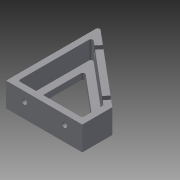
# Autodesk Inventor part: lcd_halterung_162C_links
Saved by Autodesk Inventor 2015 (Build 190159000, 159)
## iProperties
Created: 2014-11-18
Part Number: lcd_halterung_162C_links
Material: Generisch
Document SubType Name: Modeling
Designer: Zephram
Density: 1 g/cm^3
Appearance: Vorgabe
Author: Zephram
Autodesk Inventor part; units mm, degrees
ref_plane "YZ Plane" through (0, 0, 0) normal (1, 0, 0) x (0, 1, 0)
ref_plane "XZ Plane" through (0, 0, 0) normal (0, 1, 0) x (-1, 0, 0)
ref_plane "XY Plane" through (0, 0, 0) normal (0, 0, 1) x (1, 0, 0)
sketch "Skizze1" plane through (0, 0, 0) normal (0, 0, 1) x (1, 0, 0)
  line L0 (0, 0) -> (0, 46.8858)
  line L1 (0, 46.8858) -> (38, 15)
  line L2 (38, 15) -> (38, 0)
  line L3 (38, 0) -> (0, 0)
  line L4 (6.5, 32.9465) -> (6.5, 6.5)
  line L5 (6.5, 6.5) -> (31.5, 6.5)
  line L6 (31.5, 6.5) -> (31.5, 11.969)
  line L7 (31.5, 11.969) -> (6.5, 32.9465)
  dimension "d0" = 130
  dimension "d1" = 15
  dimension "d2" = 38
  dimension "d3" = 6.5
  dimension "d4" = 6.5
  dimension "d5" = 6.5
  dimension "d6" = 6.5
  constraints: 16 end point, 5 parallel, 1 perpendicular, 1 vertical
  measures "d0" angle of L2 L1
  measures "d1" distance of L1.end L2.end
  measures "d2" distance of L2.end L0.start
  measures "d3" distance between parallel lines of L3 L5
  measures "d4" distance between parallel lines of L0 L4
  measures "d5" distance between parallel lines of L1 L7
  measures "d6" distance between parallel lines of L2 L6
extrude "Extrusion1" add sketch "Skizze1" along normal blind 12
sketch "Skizze2" plane through (0, 0, 12) normal (0, 0, 1) x (1, 0, 0)
  line L0 (3, 40.4523) -> (3, 3)
  line L1 (3, 3) -> (35, 3)
  line L2 (35, 3) -> (35, 13.6011)
  line L3 (35, 13.6011) -> (3, 40.4523)
  line L4 (0, 0) -> (38, 0) projected
  line L5 (0, 46.8858) -> (0, 0) projected
  line L6 (38, 15) -> (0, 46.8858) projected
  line L7 (38, 0) -> (38, 15) projected
  dimension "d9" = 3
  dimension "d10" = 3
  dimension "d11" = 3
  dimension "d12" = 3
  constraints: 8 end point, 4 parallel, 1 horizontal, 1 perpendicular
  measures "d9" distance between parallel lines of L6 L3
  measures "d10" distance between parallel lines of L5 L0
  measures "d11" distance between parallel lines of L4 L1
  measures "d12" distance between parallel lines of L7 L2
extrude "Extrusion2" cut sketch "Skizze2" against normal blind 9 contours L3 L2 L1 L0
sketch "Skizze3" plane through (3, 3, 12) normal (0, 1, 0) x (1, 0, 0)
  line L0 (-3, 0) -> (-3, 12) projected
  line L1 (-3, 12) -> (35, 12) projected
  line L2 (35, 12) -> (35, 0) projected
  line L3 (35, 0) -> (32, 0) projected
  line L4 (32, 0) -> (0, 0) projected
  line L5 (0, 0) -> (-3, 0) projected
  line L6 (32, 0) -> (32, 9) projected
  line L7 (32, 9) -> (0, 9) projected
  line L8 (0, 9) -> (0, 0) projected
  line L9 (0, 0) -> (0, 9) projected
  line L10 (32, 0) -> (32, 9) projected
  line L11 (32, 4.5) -> (0, 4.5)
  point P0 (6, 4.5)
  point P1 (26, 4.5)
  dimension "d15" = 6
  dimension "d17" = 6
  constraints: 2 end point, 2 midpoint, 2 point on line
  measures "d15" distance of point (6, 4.5) L11.end
  measures "d17" distance of point (26, 4.5) L11.start
hole "Bohrung1" at (9, 3, 7.5) at (29, 3, 7.5) direction (0, -1, 0) diameter 2.7 depth 8 tip angle 118
fillet "Rundung1" radius 1 9 edges at (35, 13.6011, 7.5) (31.5, 11.969, 1.5) (31.5, 6.5, 1.5) (35, 3, 7.5) (6.5, 6.5, 1.5) (3, 3, 7.5) (6.5, 32.9465, 1.5) (3, 40.4523, 7.5) (0, 46.8858, 6)
sketch "Skizze4" plane through (4.6428, 39.0738, 3) normal (-0.6427876, -0.7660444, 0) x (0.7660444, -0.6427876, 0)
  line L0 (-6.0607, 9) -> (0, 9) projected
  line L1 (0, 9) -> (39.1622, 9) projected
  line L2 (39.1622, 9) -> (43.5447, 9) projected
  line L3 (43.5447, 9) -> (43.5447, -3) projected
  line L4 (43.5447, -3) -> (-6.0607, -3) projected
  line L5 (-6.0607, -3) -> (-6.0607, 9) projected
  line L6 (0, 0) -> (0, 9) projected
  line L7 (0, 0) -> (39.1622, 0) projected
  line L8 (39.1622, 0) -> (39.1622, 9) projected
  point P0 (21.5596, -3)
  point P1 (35.1622, 6.5)
  point P2 (4.1622, 6.5)
  point P3 (35.1622, 6.5)
  dimension "d26" = 2.5
  dimension "d27" = 4
  dimension "d28" = 2.5
  dimension "d29" = 35
  dimension "d30" = 4.1622
  constraints: 1 coincident
  measures "d26" distance from line of L1 point (35.162, 6.5)
  measures "d27" distance from line of L8 point (35.162, 6.5)
  measures "d28" distance from line of L1 point (4.162, 6.5)
  measures "d29" distance from line of point (4.162, 6.5) L8
  measures "d30" distance from line of L6 point (4.162, 6.5)
hole "Bohrung2" at (31.5786, 16.472, 9.5) at (7.8312, 36.3984, 9.5) direction (0.6427876, 0.7660444, 0) diameter 2.5 depth 8 tip angle 118
sketch "Skizze5" plane through (38, 15, 12) normal (0.6427876, 0.7660444, 0) x (0.7660444, -0.6427876, 0)
  circle A0 centre (-5.8652, 2.5) radius 1.25 projected
  line L0 (-4.6152, 2.5) -> (-4.6152, 0)
  line L1 (-19.4679, 0) -> (9.6418, 0) projected
  line L2 (-7.1152, 2.5) -> (-7.1152, 0)
  circle A1 centre (-36.8652, 2.5) radius 1.25 projected
  line L3 (-35.6152, 2.5) -> (-35.6152, 0)
  line L4 (-41.0274, 0) -> (-1.8652, 0) projected
  line L5 (-38.1152, 2.5) -> (-38.1152, 0)
  point P0 (-19.4679, 12)
  constraints: 8 end point, 4 point on circle, 4 point on line, 4 tangent, 3 parallel, 1 vertical
extrude "Extrusion3" cut sketch "Skizze5" against normal blind 4.5 contours L0 L1 L2 A0 | L3 L4 L5 A1
